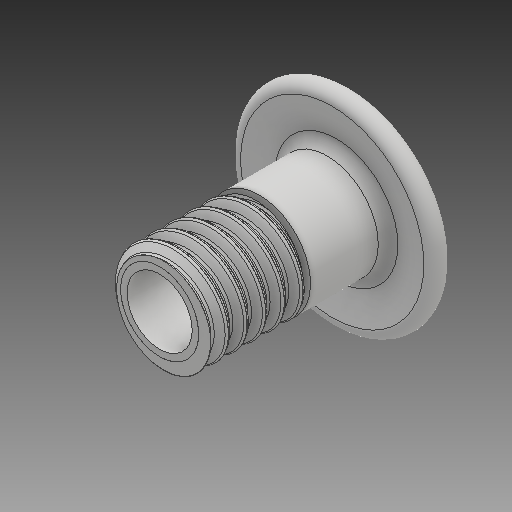
# Autodesk Inventor part: Kabelzugentlastung
Saved by Autodesk Inventor 2018.2 (Build 222227000, 227)
## iProperties
Created: 2018-01-25
Part Number: Kabelzugentlastung
Material: Generisch
Document SubType Name: Modeling
Designer: JochenAlt
Density: 1 g/cm^3
Appearance: Vorgabe
Author: JochenAlt
Autodesk Inventor part; units mm, degrees
ref_plane "YZ Plane" through (0, 0, 0) normal (1, 0, 0) x (0, 1, 0)
ref_plane "XZ Plane" through (0, 0, 0) normal (0, 1, 0) x (-1, 0, 0)
ref_plane "XY Plane" through (0, 0, 0) normal (0, 0, 1) x (1, 0, 0)
sketch "Skizze1" plane through (0, 0, 0) normal (0, 0, 1) x (1, 0, 0)
  line L0 (0, 77.3285) -> (0, -12.8881) construction
  line L1 (-9.5494, 0) -> (57.2964, 0) construction
  arc A0 (10.1613, 62.1751) -> (4.032, 62.8708) centre (0, 0) ccw
  line L2 (5.5, 62.9404) -> (5.5, 63.1904)
  line L3 (4.25, 64.4404) -> (4.25, 64.4404)
  line L4 (5.5, 59.6469) -> (5.5, 41.6469)
  line L5 (3.5, 62.3719) -> (3.5, 41.6469)
  line L6 (5.5, 41.6469) -> (3.5, 41.6469)
  arc A1 (9.8387, 60.2013) -> (6.6083, 60.641) centre (0, 0) ccw
  arc A2 (6.6083, 60.641) -> (5.5, 59.6469) centre (6.5, 59.6469) ccw
  arc A3 (4.032, 62.8708) -> (3.5, 62.3719) centre (4, 62.3719) ccw
  arc A4 (9.8387, 60.2013) -> (10.1613, 62.1751) centre (10, 61.1882) ccw
  arc A5 (9.8387, 60.2013) -> (6.6083, 60.641) centre (0, 0) ccw
  point P0 (4.8231, 61.4229)
  point P1 (4.8231, 61.4229)
  point P2 (3.5, 62.9027)
  point P3 (9.5, 60.2557)
  point P4 (47.747, 41.6469)
  dimension "d551" = 9.5
  dimension "d552" = 1
  dimension "d553" = 18
  dimension "d573" = 0.5
  dimension "d607" = 10
  dimension "d608" = 61
  dimension "d609" = 3.5
  dimension "d610" = 5.5
  constraints: 14 point on circle, 10 end point, 6 centre point, 6 tangent, 4 coincident, 2 horizontal, 2 point on line, 2 vertical, 1 collinear, 2 other
  measures "d551" distance from line of point (9.5, 60.256) L0
  measures "d552" radius of A2
  measures "d553" distance from line of L6 A2.centre
  measures "d573" radius of A3
  measures "d607" distance from line of A4.centre L0
  measures "d608" radius of A1
  measures "d609" distance between parallel lines of L0 L5
  measures "d610" distance between parallel lines of L0 L4
revolve "Umdrehung58" add sketch "Skizze1" angle 360 about axis through (0, 0, 0) along (0, -1, 0)
thread "Gewinde7" size "M16x2" class "6g" standard "ANSI Metric M Profile" length 18 offset 4
sketch "Skizze93" plane through (0, 56.0492, 0) normal (1, 0, 0) x (0, 0, 1)
  line L0 (5.5, 3.6885) -> (5.5, 18)
  line L1 (5.5, 18) -> (4.1948, 18)
  line L2 (4.1948, 18) -> (4.1948, 3.6885)
  line L3 (4.1948, 3.6885) -> (5.5, 3.6885)
  line L4 (0, 0.8262) -> (0, 20.8623) projected
  constraints: 8 end point
revolve "Umdrehung59" cut sketch "Skizze93" angle 360 about axis through (0, 56.0492, 0) along (0, -1, 0)
sketch "Skizze94" plane through (0, 56.0492, 0) normal (1, 0, 0) x (0, 0, 1)
  line L0 (5.5, 3.6885) -> (5.5, 14.4024)
  line L1 (5.5, 14.4024) -> (4.1948, 14.4024)
  line L2 (4.1948, 14.4024) -> (4.1948, 3.6885)
  line L3 (4.1948, 3.6885) -> (5.5, 3.6885)
  line L4 (0, 1.3457) -> (0, 17.7451) projected
  line L5 (-5.5, 3.6885) -> (5.5, 3.6885) construction
  line L6 (4.1948, 14.4024) -> (-4.1948, 14.4024) construction
  point P0 (4.8474, 3.6885)
  point P1 (4.8474, 14.4024)
  constraints: 8 end point, 2 midpoint, 2 point on line
revolve "Umdrehung60" add sketch "Skizze94" angle 360 about axis through (0, 56.0492, 0) along (0, -1, 0) separate body
sketch "Skizze92" plane through (0, 56.0492, 0) normal (-1, 0, 0) x (0, -1, 0)
  line L0 (-1.2458, -4.7161) -> (-1.0001, -4.7161) construction
  line L1 (0.2456, -5.379) -> (-0.0001, -5.6992) construction
  line L2 (-2.0001, -5.6992) -> (-2.2458, -5.379) construction
  line L3 (-0.7544, -4.7161) -> (-1.0001, -4.396) construction
  line L4 (-1.0001, -4.396) -> (-1.2458, -4.7161) construction
  line L5 (-2.0001, -5.6992) -> (-1.7544, -5.379) construction
  line L6 (-0.7544, -4.7161) -> (-0.2458, -5.379)
  line L7 (-2.2458, -5.379) -> (-1.7544, -5.379) construction
  arc A0 (-2.2458, -5.379) -> (-2.0001, -5.5002) centre (-2.0001, -5.1905) ccw construction
  line L8 (0.2456, -5.379) -> (-0.2458, -5.379) construction
  line L9 (-2.0001, -5.6992) -> (-2.0001, -5.379) construction
  line L10 (-0.0001, -5.6992) -> (-0.0001, -5.379) construction
  line L11 (-1.0001, -4.396) -> (-1.0001, -4.595) construction
  line L12 (-2.0001, -5.5002) -> (-0.0001, -5.5002)
  arc A1 (-2.0001, -5.5002) -> (-1.7544, -5.379) centre (-2.0001, -5.1905) ccw
  line L13 (-0.2458, -5.379) -> (-0.0001, -5.6992) construction
  line L14 (-1.7544, -5.379) -> (-1.2458, -4.7161)
  line L15 (-0.0001, -0.0002) -> (-0.0001, 0.0177)
  line L16 (-0.0001, 0.0177) -> (-0.0001, -0.0002)
  line L17 (-0.0001, -0.0002) -> (0.0334, -0.0002)
  arc A2 (-0.2458, -5.379) -> (-0.0001, -5.5002) centre (-0.0001, -5.1905) ccw
  arc A3 (-0.0001, -5.5002) -> (0.2456, -5.379) centre (-0.0001, -5.1905) ccw construction
  arc A4 (-1.0001, -4.595) -> (-1.2458, -4.7161) centre (-1.0001, -4.9046) ccw
  arc A5 (-0.7544, -4.7161) -> (-1.0001, -4.595) centre (-1.0001, -4.9046) ccw
  line L18 (-1.0001, -4.595) -> (-1.0001, -4.7161) construction
  line L19 (-1.0001, -4.7161) -> (-0.7544, -4.7161) construction
  dimension "d588" = 75
  dimension "d589" = 0.3202
  dimension "d590" = 0.3202
  dimension "Skizze92_ThreadOffset" = 0
  dimension "Skizze92_MajorRadius" = 5.5
  dimension "d593" = 2
  dimension "Skizze92_MinorRadius" = 4.5948
  constraints: 40 end point, 12 point on circle, 10 parallel, 8 tangent, 6 centre point, 6 collinear, 2 midpoint, 2 point on line, 1 horizontal, 1 perpendicular, 3 other
  measures "d588" angle of L6 L14
  measures "d589" distance of L3.end L0.end
  measures "d590" distance of L1.end L10.end
  measures "Skizze92_ThreadOffset" distance between parallel lines of L15 L10
  measures "Skizze92_MajorRadius" distance from line of L12 L15.start
  measures "d593" distance from line of L1.end L9
  measures "Skizze92_MinorRadius" distance edge to line of A5 L17
coil "Spirale29" sketch "Skizze92" operation cut axis through (0, 56.0492, 0) along (0, -1, 0) pitch 2.002 turns 10.989011 hand right bodies 2
equation "\"d26\" = 60deg"
equation "\"Skizze2_Pitch\" = 1"
equation "\"d47\" = 60deg"
equation "\"Skizze5_Pitch\" = 2"
equation "\"d70\" = 60deg"
equation "\"Skizze8_Pitch\" = 2"
equation "\"d90\" = 60deg"
equation "\"Skizze11_Pitch\" = 2"
equation "\"d111\" = 60deg"
equation "\"Skizze14_Pitch\" = 2.54"
equation "\"d130\" = 60deg"
equation "\"Skizze17_Pitch\" = 2"
equation "\"d149\" = 60deg"
equation "\"Skizze20_Pitch\" = 1.33684"
equation "\"d168\" = 60deg"
equation "\"Skizze23_Pitch\" = 1.3"
equation "\"d187\" = 60deg"
equation "\"Skizze26_Pitch\" = 1.33684"
equation "\"d206\" = 60deg"
equation "\"Skizze29_Pitch\" = 1.33684"
equation "\"d225\" = 60deg"
equation "\"Skizze32_Pitch\" = 2.6"
equation "\"d244\" = 60deg"
equation "\"Skizze35_Pitch\" = 1.5"
equation "\"d263\" = 60deg"
equation "\"Skizze38_Pitch\" = 2.54"
equation "\"d282\" = 60deg"
equation "\"Skizze42_Pitch\" = 2.30909"
equation "\"d301\" = 60deg"
equation "\"Skizze46_Pitch\" = 3"
equation "\"d320\" = 60deg"
equation "\"Skizze49_Pitch\" = 2"
equation "\"d339\" = 60deg"
equation "\"Skizze53_Pitch\" = 1"
equation "\"d358\" = 60deg"
equation "\"Skizze56_Pitch\" = 2"
equation "\"d383\" = 60deg"
equation "\"Skizze59_Pitch\" = 1.5"
equation "\"d402\" = 60deg"
equation "\"Skizze62_Pitch\" = 1.5"
equation "\"d421\" = 60deg"
equation "\"Skizze65_Pitch\" = 5"
equation "\"d440\" = 60deg"
equation "\"Skizze68_Pitch\" = 5"
equation "\"d459\" = 60deg"
equation "\"Skizze71_Pitch\" = 3.6"
equation "\"d478\" = 60deg"
equation "\"Skizze74_Pitch\" = 2.2"
equation "\"d497\" = 60deg"
equation "\"Skizze77_Pitch\" = 2.2"
equation "\"d516\" = 60deg"
equation "\"Skizze80_Pitch\" = 2"
equation "\"d535\" = 60deg"
equation "\"Skizze83_Pitch\" = 2"
equation "\"d561\" = 60deg"
equation "\"Skizze86_Pitch\" = 2"
equation "\"d595\" = 60deg"
equation "\"Skizze92_Pitch\" = 2"
